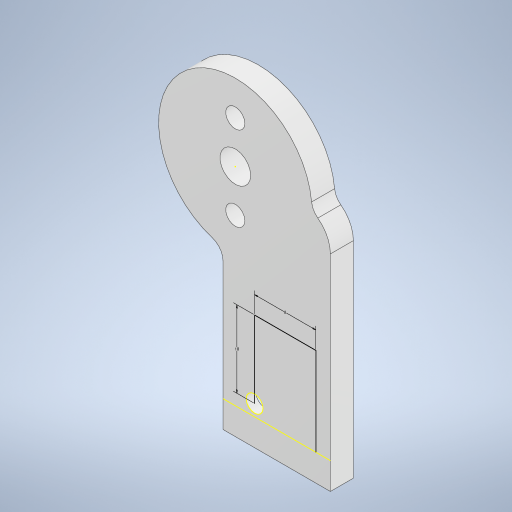
# Autodesk Inventor part: cutter_board_claws_endeffector_8_5_rotary-blade
Saved by Autodesk Inventor 2024 (Build 280153000, 153)
## iProperties
Created: 2025-06-01
Part Number: cutter_board_claws_endeffector_8_5_rotary-blade
Material: ABS プラスチック
Document SubType Name: Modeling
Designer: 1412z
Density: 1.06 g/cm^3
Appearance: 滑らか - 白
Author: 1412z
Autodesk Inventor part; units mm, degrees
ref_plane "YZ Plane" through (0, 0, 0) normal (1, 0, 0) x (0, 1, 0)
ref_plane "XZ Plane" through (0, 0, 0) normal (0, 1, 0) x (-1, 0, 0)
ref_plane "XY Plane" through (0, 0, 0) normal (0, 0, 1) x (1, 0, 0)
sketch "スケッチ1" plane through (0, 0, 0) normal (0, 0, 1) x (1, 0, 0)
  circle A0 centre (0, 0) radius 10
  line L0 (0, 0) -> (12.4, 0)
  line L1 (12.4, 0) -> (12.4, -45)
  line L2 (12.4, -45) -> (-1.6, -45)
  line L3 (-1.6, -45) -> (-1.6, 0)
  circle A1 centre (2.5, -25.5) radius 1.1
  circle A2 centre (2.5, -32) radius 1.7
  circle A3 centre (2.5, -42) radius 1.7
  circle A4 centre (0, 0) radius 5.5
  circle A5 centre (0, 5.5) radius 1.25
  circle A6 centre (0, -5.5) radius 1.25
  circle A7 centre (0, 0) radius 2
  line L4 (0, 0) -> (0, -45)
  line L5 (2.5, -25.5) -> (12.4, -25.5)
  point P0 (7.5, -6.6144)
  point P1 (-1.6, -9.8712)
  point P2 (10, 0)
  dimension "d0" = 20
  dimension "d3" = 12.4
  dimension "d4" = 45
  dimension "d5" = 14
  dimension "d6" = 2.2
  dimension "d7" = 3.4
  dimension "d8" = 3.4
  dimension "d9" = 11
  dimension "d10" = 2.5
  dimension "d11" = 2.5
  dimension "d12" = 4
  dimension "d16" = 2.5
  dimension "d17" = 2.5
  dimension "d18" = 2.5
  dimension "d19" = 9.9
  dimension "d37" = 25.5
  constraints: 12 end point, 8 centre point, 4 perpendicular, 3 coincident, 2 horizontal, 2 point on circle, 2 point on line
  measures "d0" diameter of A0
  measures "d3" distance of L0.start L0.end
  measures "d4" distance of L0.end L1.end
  measures "d5" distance of L1.end L2.end
  measures "d6" diameter of A1
  measures "d7" diameter of A2
  measures "d8" diameter of A3
  measures "d9" diameter of A4
  measures "d10" diameter of A5
  measures "d11" diameter of A6
  measures "d12" diameter of A7
  measures "d16" distance from line of L4 L5.start
  measures "d17" distance from line of L4 A2.centre
  measures "d18" distance from line of L4 A3.centre
  measures "d19" distance of L5.start L5.end
  measures "d37" distance from line of L0 L5.start
extrude "押し出し1" add sketch "スケッチ1" along normal blind 3 contours L0 A4 A5 L3 A0 | L0 L1 L2 L4 A0 | A0 L4 A6 A4 L0 | L3 A4 A6 L4 A0 | A0 L4 L2 L3 | A4 A6 L4 A7 L0 | L0 A7 L3 A4 A5 | L3 A7 L4 A6 A4
fillet "フィレット1" radius 2 1 edges at (-1.6, -9.8712, 1.5)
fillet "フィレット2" radius 4 1 edges at (12.4, 0, 1.5)
fillet "フィレット3" radius 2 1 edges at (10, 0, 1.5)
sketch "スケッチ2" plane through (0, 0, 3) normal (0, 0, 1) x (1, 0, 0)
  line L0 (12.4, -45) -> (12.4, -3.6661) projected
  line L1 (12.4, -45) -> (12.4, -27)
  line L2 (12.4, -27) -> (-1.6, -27)
  line L3 (-1.6, -11.4473) -> (-1.6, -45) projected
  line L4 (-1.6, -27) -> (-1.6, -45)
  line L5 (-1.6, -45) -> (12.4, -45) projected
  line L6 (-1.6, -45) -> (12.4, -45)
  point P0 (0, 0)
  dimension "d22" = 18
  constraints: 8 end point, 2 point on line, 1 collinear, 1 perpendicular, 1 vertical
  measures "d22" distance of L0.start L1.end
extrude "押し出し2" cut sketch "スケッチ2" against normal blind 10
sketch "スケッチ3" plane through (0, 0, 3) normal (0, 0, 1) x (1, 0, 0)
  circle A0 centre (2.5, -25.5) radius 1.1 projected
  line L0 (2.5, -25.5) -> (2.5, -15.5)
  line L1 (2.5, -15.5) -> (10.5, -15.5)
  line L2 (10.5, -15.5) -> (10.5, -27)
  line L3 (-1.6, -27) -> (12.4, -27) projected
  point P0 (0, 0)
  dimension "d25" = 10
  dimension "d26" = 8
  constraints: 6 end point, 2 vertical, 1 perpendicular, 1 point on line
  measures "d25" distance of L0.start L0.end
  measures "d26" distance of L0.end L1.end
sketch "スケッチ5" plane through (-1.6, -27, 3) normal (0, -1, 0) x (1, 0, 0)
  line L0 (0, -3) -> (0, 0) projected
  line L1 (0, -1.5) -> (0, -1.3)
  line L2 (0, -1.3) -> (12.1, -1.3)
  line L3 (12.1, -1.3) -> (12.1, -1.7)
  line L4 (12.1, -1.7) -> (0, -1.7)
  line L5 (0, -1.7) -> (0, -1.5)
  point P0 (1.6, -3)
  point P1 (0, -1.7)
  dimension "d32" = 0.2
  dimension "d33" = 12.1
  dimension "d34" = 0.4
  constraints: 10 end point, 4 perpendicular, 2 point on line, 1 midpoint
  measures "d32" distance of L1.start L1.end
  measures "d33" distance of L1.end L2.end
  measures "d34" distance of L2.end L3.end
extrude "押し出し4" cut sketch "スケッチ5" against normal blind 11.5
sketch "スケッチ6" plane through (-1.6, -27, 3) normal (0, -1, 0) x (1, 0, 0)
  line L0 (12.3614, 0) -> (14, 0) projected
  line L1 (0, -3) -> (0, 0) projected
  line L2 (14, 0) -> (0, 0)
  line L3 (0, -1.3) -> (12.1, -1.3) projected
  line L4 (0, 0) -> (0, -1.3)
  line L5 (12.1, -1.3) -> (12.1, -1.7) projected
  line L6 (0, -1.3) -> (12.1, -1.3)
  line L7 (12.1, -1.7) -> (0, -1.7) projected
  line L8 (12.1, -1.3) -> (12.1, -1.7)
  line L9 (12.1, -1.7) -> (0, -1.7)
  line L10 (0, -1.7) -> (0, -3)
  line L11 (0, -3) -> (14, -3)
  line L12 (14, -3) -> (14, 0)
  point P0 (1.6, -3)
  constraints: 16 end point, 6 perpendicular, 1 collinear, 1 horizontal
extrude "押し出し5" add sketch "スケッチ6" along normal blind 3.5 contours L0 L12 L11 L1 L7 L5 L3 L2
sketch "スケッチ7" plane through (0, 0, 0) normal (0, 0, -1) x (-1, 0, 0)
  line L0 (1.6, -11.4473) -> (1.6, -30.5) projected
  line L1 (1.6, -30.5) -> (1.6, -15.5)
  line L2 (-10.5, -15.5) -> (1.6, -15.5) projected
  line L3 (1.6, -15.5) -> (-10.5, -15.5)
  line L4 (-10.5, -15.5) -> (-10.5, -30.5)
  line L5 (-10.5, -30.5) -> (1.6, -30.5)
  point P0 (0, 0)
  constraints: 8 end point, 2 perpendicular, 1 collinear
extrude "押し出し6" cut sketch "スケッチ7" against normal blind 1.5
